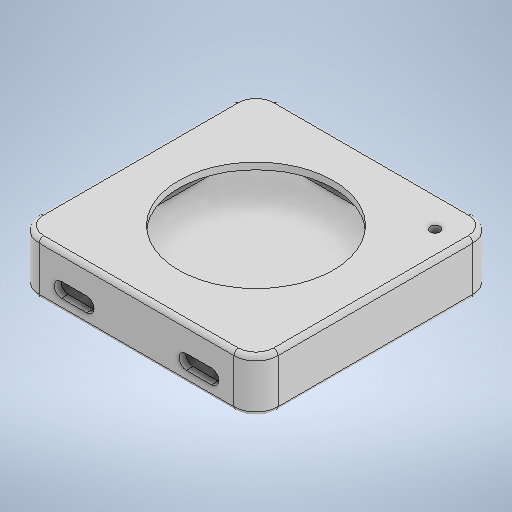
# Autodesk Inventor part: Box
Saved by Autodesk Inventor 2026 (Build 300175050, 175E)
## iProperties
Created: 2025-07-10
Part Number: Box
Material: Generic
Document SubType Name: Modeling
Designer: Jochen Alt
Density: 1 g/cm^3
Appearance: Default
Author: Jochen Alt
Autodesk Inventor part; units mm, degrees
ref_plane "YZ Plane" through (0, 0, 0) normal (1, 0, 0) x (0, 1, 0)
ref_plane "XZ Plane" through (0, 0, 0) normal (0, 1, 0) x (-1, 0, 0)
ref_plane "XY Plane" through (0, 0, 0) normal (0, 0, 1) x (1, 0, 0)
sketch "Sketch1" plane through (0, 0, 0) normal (0, 0, 1) x (1, 0, 0)
  line L0 (0, 37.8) -> (0, -37.8) construction
  line L1 (-37.8, 0) -> (37.8, 0) construction
  line L2 (-27, 27) -> (27, 27)
  line L3 (27, 27) -> (27, -27)
  line L4 (27, -27) -> (-27, -27)
  line L5 (-27, -27) -> (-27, 27)
  circle A0 centre (0, 0) radius 17.5
  dimension "d1" = 54
  dimension "d2" = 54
  dimension "d25" = 35
  constraints: 8 end point, 2 parallel, 1 centre point, 1 coincident, 1 horizontal, 1 perpendicular, 2 other
  measures "d1" distance between parallel lines of L3 L5
  measures "d2" distance between parallel lines of L4 L2
  measures "d25" diameter of A0
extrude "Extrusion1" add sketch "Sketch1" along normal blind 12 contours L2 L3 L4 L5 | A0
fillet "Fillet1" radius 5 4 edges at (-27, -27, 6) (27, -27, 6) (27, 27, 6) (-27, 27, 6)
fillet "Fillet2" radius 1 16 edges at (-25.5355, 25.5355, 12) (-27, 0, 12) (-25.5355, -25.5355, 12) (0, -27, 12) (25.5355, -25.5355, 12) (27, 0, 12) (25.5355, 25.5355, 12) (0, 27, 12) (-25.5355, 25.5355, 0) (-27, 0, 0) (-25.5355, -25.5355, 0) (0, -27, 0) (25.5355, -25.5355, 0) (27, 0, 0) (25.5355, 25.5355, 0) (0, 27, 0)
shell "Shell2" thickness 1.5 removed faces 0
sketch "USBPort" plane through (0, 0, 0) normal (0, 1, 0) x (-1, 0, 0)
  line L0 (16.95, 4.4) -> (11.25, 4.4) construction
  line L1 (16.95, 2.75) -> (11.25, 2.75)
  line L2 (11.25, 6.05) -> (16.95, 6.05)
  arc A0 (16.95, 2.75) -> (16.95, 6.05) centre (16.95, 4.4) ccw
  arc A1 (11.25, 6.05) -> (11.25, 2.75) centre (11.25, 4.4) ccw
  line L3 (-27.9, 0) -> (34.4, 0) construction
  line L4 (0, -2.1) -> (0, 12.6) construction
  circle A2 centre (19, 7) radius 1
  line L5 (-16.95, 2.75) -> (-11.25, 2.75)
  line L6 (-11.25, 6.05) -> (-16.95, 6.05)
  arc A3 (-16.95, 6.05) -> (-16.95, 2.75) centre (-16.95, 4.4) ccw
  arc A4 (-11.25, 2.75) -> (-11.25, 6.05) centre (-11.25, 4.4) ccw
  line L7 (25.5, 1.5) -> (25.5, 10.5) projected
  line L8 (27, 11) -> (27, 1) projected
  line L9 (22, 12) -> (26, 12) projected
  point P0 (0, 0)
  point P1 (14.1, 4.4)
  point P2 (9.6, 4.4)
  point P3 (18.6, 4.4)
  point P4 (14.1, 6.05)
  dimension "d20" = 2
  dimension "d33" = 9
  dimension "d34" = 3.3
  dimension "d35" = 6.9
  dimension "d62" = 8
  dimension "d63" = 5
  constraints: 12 end point, 10 point on circle, 6 symmetric about line, 5 centre point, 4 tangent, 2 midpoint, 1 horizontal, 1 parallel, 2 other
  measures "d20" diameter of A2
  measures "d33" distance of point (9.6, 4.4) point (18.6, 4.4)
  measures "d34" distance from line of L1 point (14.1, 6.05)
  measures "d35" distance from line of point (18.6, 4.4) L7
  measures "d62" distance from line of A2.centre L8
  measures "d63" distance from line of A2.centre L9
extrude "USB Port" cut sketch "USBPort" against normal up to next contours L1 A1 L2 A0 | A3 L6 A4 L5
extrude "Extrusion5" cut sketch "USBPort" along normal up to next contours A2
extrude "Extrusion6" cut sketch "Sketch1" against normal blind 5 from surface at 12 contours A0
sketch "LED" plane through (0, 0, 0) normal (0, 0, 1) x (1, 0, 0)
  line L0 (0, 37.8) -> (0, -37.8) construction
  line L1 (-37.8, 0) -> (37.8, 0) construction
  line L2 (-27, 27) -> (27, 27) construction
  line L3 (-27, -27) -> (-27, 27) construction
  line L4 (27, -27) -> (-27, -27) construction
  line L5 (27, 27) -> (27, -27) construction
  line L6 (-22, -25.5) -> (22, -25.5) projected
  line L7 (21.1602, 3.5249) -> (17.1869, 3.9858)
  line L8 (17.1869, 3.9858) -> (17.6478, 7.9591)
  line L9 (17.6478, 7.9591) -> (21.6211, 7.4982)
  line L10 (21.6211, 7.4982) -> (21.1602, 3.5249)
  line L11 (21.1602, 3.5249) -> (17.6478, 7.9591) construction
  line L12 (20.4552, 6.5747) -> (17.1869, 3.9858) construction
  circle A0 centre (21, 19.5) radius 1.1
  line L13 (19.3371, 18.1828) -> (19.6828, 21.1629)
  line L14 (19.6828, 21.1629) -> (22.6629, 20.8172) construction
  line L15 (22.6629, 20.8172) -> (22.3172, 17.8371)
  line L16 (22.3172, 17.8371) -> (19.6828, 21.1629) construction
  line L17 (19.3371, 18.1828) -> (22.6629, 20.8172) construction
  line L18 (21, 19.5) -> (19.404, 5.742) construction
  line L19 (-18, 25.5) -> (-20, 25.5) construction
  line L20 (-22, 25.5) -> (22, 25.5) construction
  line L21 (-22, 25.5) -> (22, 25.5) construction
  line L22 (-25.5, -22) -> (-25.5, 22) construction
  line L23 (-25.5, 22) -> (-25.5, -22) construction
  circle A1 centre (19.404, 5.742) radius 1.5 construction
  circle A2 centre (19.404, 5.742) radius 1.5 construction
  line L24 (19.6828, 21.1629) -> (19.9133, 23.1495)
  line L25 (19.9133, 23.1495) -> (22.8933, 22.8038)
  line L26 (22.8933, 22.8038) -> (22.6629, 20.8172)
  line L27 (19.7405, 21.6595) -> (22.7205, 21.3138)
  line L28 (19.347, 18.2681) -> (22.327, 17.9224)
  line L29 (22.8933, 22.8038) -> (23.2061, 25.5)
  line L30 (20.186, 25.5) -> (19.9133, 23.1495)
  line L31 (23.2061, 25.5) -> (20.186, 25.5)
  point P0 (0, 0)
  point P1 (-17, 25.5)
  point P2 (-19, 25.5)
  point P3 (39.0896, 25.5)
  dimension "d37" = 4
  dimension "d38" = 2.2
  dimension "d40" = 3
  dimension "d56" = 6
  dimension "d58" = 2
  dimension "d59" = 0.5
  dimension "d60" = 1.4142
  dimension "d64" = 6
  constraints: 40 end point, 8 perpendicular, 7 point on line, 5 midpoint, 4 coincident, 4 collinear, 4 parallel, 2 centre point, 1 other
  measures "d37" distance of L8.end L9.end
  measures "d38" diameter of A0
  measures "d40" distance of L13.end L14.end
  measures "d56" distance from line of L20 point (21, 19.5)
  measures "d58" distance of L25.end L14.end
  measures "d59" distance between parallel lines of L14 L27
  measures "d60" distance from line of A0.centre L28
  measures "d64" distance from line of L5 A0.centre
extrude "Extrusion8" add sketch "LED" against normal blind 4 from surface at 10.5 contours L7 L8 L9 L10
chamfer "Chamfer1" distance 4 angle 45 1 edges at (19.6345, 7.7287, 6.5)
extrude "Extrusion9" add sketch "LED" against normal blind 4 from surface at 10.5 separate body contours A0 | L13 L24 L27 L26 L15 L28 | L24 L25 L26 L27 | L30 L31 L29 L25
chamfer "Chamfer2" distance 4 angle 45 1 edges at (20.837, 18.0952, 10.5)
combine bodies "Combine1" operation type add bodies to combine 2 1
extrude "Extrusion10" cut sketch "LED" against normal blind 2 from surface at 12 contours A0 bodies 2
equation "\"d2\" = d1"
equation "\"d56\" = d41"
equation "\"d60\" = 0.353553 * d37"
equation "\"d64\" = d56"
equation "\"d41\" = 6"
body "Solid2"
